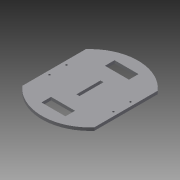
# Autodesk Inventor part: base
Saved by Autodesk Inventor 2015 (Build 190159000, 159)
## iProperties
Created: 2014-10-23
Part Number: base
Material: Generic
Document SubType Name: Modeling
Designer: Colin
Density: 1 g/cm^3
Appearance: Default
Author: Colin
Autodesk Inventor part; units mm, degrees
ref_plane "YZ Plane" through (0, 0, 0) normal (1, 0, 0) x (0, 1, 0)
ref_plane "XZ Plane" through (0, 0, 0) normal (0, 1, 0) x (-1, 0, 0)
ref_plane "XY Plane" through (0, 0, 0) normal (0, 0, 1) x (1, 0, 0)
sketch "Sketch6" plane through (0, 0, 0) normal (0, 1, 0) x (-1, 0, 0)
  circle A0 centre (0, 0) radius 50.8
  line L0 (38.1, 0) -> (38.1, 33.601)
  line L1 (-38.1, 0) -> (-38.1, 33.601)
  line L2 (38.1, 0) -> (38.1, -33.601)
  line L3 (-38.1, 0) -> (-38.1, -33.601)
  line L4 (38.1, -33.601) -> (-38.1, -33.601) construction
  line L5 (38.1, 33.601) -> (-38.1, 33.601) construction
  line L6 (12.7, -38.6842) -> (-12.7, -38.6842)
  line L7 (-12.7, -38.6842) -> (-12.7, -28.5242)
  line L8 (-12.7, -28.5242) -> (12.7, -28.5242)
  line L9 (12.7, -28.5242) -> (12.7, -38.6842)
  line L10 (12.7, 28.5242) -> (-12.7, 28.5242)
  line L11 (-12.7, 28.5242) -> (-12.7, 38.6842)
  line L12 (-12.7, 38.6842) -> (12.7, 38.6842)
  line L13 (12.7, 38.6842) -> (12.7, 28.5242)
  line L14 (0, -33.601) -> (0, 33.601) construction
  line L15 (33.859, -33.601) -> (33.859, 33.601) construction
  circle A1 centre (33.859, -9.0011) radius 1.016
  circle A2 centre (33.859, 8.9989) radius 1.016
  circle A3 centre (-33.859, -9.0011) radius 1.016
  circle A4 centre (-33.859, 8.9989) radius 1.016
  point P0 (50.8, 0)
  point P1 (-50.8, 0)
  point P2 (0, -50.8)
  dimension "d9" = 101.6
  dimension "d10" = 12.7
  dimension "d11" = 12.7
  dimension "d14" = 25.4
  dimension "d15" = 10.16
  dimension "d16" = 25.4
  dimension "d17" = 25.4
  dimension "d18" = 25.4
  dimension "d19" = 10.16
  dimension "d20" = 57.0484
  dimension "d21" = 12.1158
  dimension "d31" = 4.241
  dimension "d32" = 18
  dimension "d33" = 24.5999
  dimension "d34" = 2.032
  dimension "d35" = 2.032
  constraints: 32 end point, 5 parallel, 4 centre point, 4 perpendicular, 4 point on line, 2 horizontal, 2 midpoint, 2 symmetric about line, 1 coincident, 1 vertical, 11 other
  measures "d10" distance of point (50.8, 0) L0.start
  measures "d11" distance of point (-50.8, 0) L1.start
  measures "d14" distance of L6.start L6.end
  measures "d15" distance of L8.end L6.start
  measures "d16" distance between parallel lines of L2 L9
  measures "d17" distance between parallel lines of L0 L13
  measures "d18" distance of L10.start L10.end
  measures "d19" distance of L12.end L10.start
  measures "d20" distance between parallel lines of L8 L10
  measures "d21" distance from line of point (0, -50.8) L6
  measures "d31" distance between parallel lines of L2 L15
  measures "d32" distance of A1.centre A2.centre
  measures "d33" distance from line of L4 A1.centre
  measures "d34" diameter of A1
  measures "d35" diameter of A2
extrude "Extrusion6" add sketch "Sketch6" along normal blind 3.175 contours L0 L2 A0 L3 L1
sketch "Sketch7" plane through (0, 3.175, 0) normal (0, 1, 0) x (1, 0, 0)
  line L0 (12.7, 28.5242) -> (-12.7, 28.5242) construction
  line L1 (0, 28.5242) -> (0, -28.5242) construction
  line L2 (-12.7, -28.5242) -> (12.7, -28.5242) construction
  line L3 (-1.5875, 12.7) -> (1.5875, 12.7)
  line L4 (1.5875, 12.7) -> (1.5875, -12.7)
  line L5 (1.5875, -12.7) -> (-1.5875, -12.7)
  line L6 (-1.5875, -12.7) -> (-1.5875, 12.7)
  line L7 (-38.1, 33.601) -> (-38.1, -33.601) projected
  point P0 (0, 0)
  dimension "d38" = 3.175
  dimension "d39" = 25.4
  dimension "d40" = 15.8242
  dimension "d41" = 36.5125
  constraints: 10 end point, 2 midpoint, 2 parallel, 1 horizontal, 1 perpendicular
  measures "d38" distance of L3.start L3.end
  measures "d39" distance of L5.end L3.start
  measures "d40" distance between parallel lines of L0 L3
  measures "d41" distance between parallel lines of L7 L6
extrude "Extrusion7" cut sketch "Sketch7" against normal through all
equation "\"d35\" = d34"
body "Solid6"
